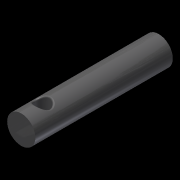
# Autodesk Inventor part: Winch Pin
Saved by Autodesk Inventor 2014 SP1 (Build 180222100, 222)
## iProperties
Created: 2014-01-20
Part Number: Winch Pin
Material: Steel
Document SubType Name: Modeling
Designer: Rauhul Varma
Mass: 7.30664 g
Surface Area: 7.18159 cm^2
Volume: 0.930782 cm^3
Density: 7.85 g/cm^3
Appearance: Steel
Author: Rauhul Varma
Autodesk Inventor part; units mm, degrees
ref_plane "YZ Plane" through (0, 0, 0) normal (1, 0, 0) x (0, 1, 0)
ref_plane "XZ Plane" through (0, 0, 0) normal (0, 1, 0) x (-1, 0, 0)
ref_plane "XY Plane" through (0, 0, 0) normal (0, 0, 1) x (1, 0, 0)
sketch "Sketch1" plane through (0, 0, 0) normal (0, 0, 1) x (1, 0, 0)
  circle A0 centre (0, 0) radius 3.175
  dimension "d0" = 6.35
  constraints: 1 centre point, 1 coincident
  measures "d0" diameter of A0
extrude "Extrusion1" add sketch "Sketch1" along normal blind 30.9563
sketch "Sketch2" plane through (0, 0, 0) normal (0, 1, 0) x (-1, 0, 0)
  line L0 (3.175, 30.9563) -> (-3.175, 30.9563) projected
  line L1 (-3.175, 0) -> (3.175, 0) projected
  line L2 (0, 0) -> (0, 30.9563) construction
  circle A0 centre (0, 26.1938) radius 1.5875
  dimension "d4" = 3.175
  dimension "d5" = 4.7625
  constraints: 2 end point, 1 centre point, 1 midpoint, 1 point on line
  measures "d4" diameter of A0
  measures "d5" distance from line of L0 A0.centre
extrude "Extrusion2" cut sketch "Sketch2" along normal through all both and the other way through all
fillet "Fillet2" radius 0.2977 2 edges at (1.5875, 2.7496, 26.1894) (1.5875, -2.7496, 26.1894)
body "Solid1"
